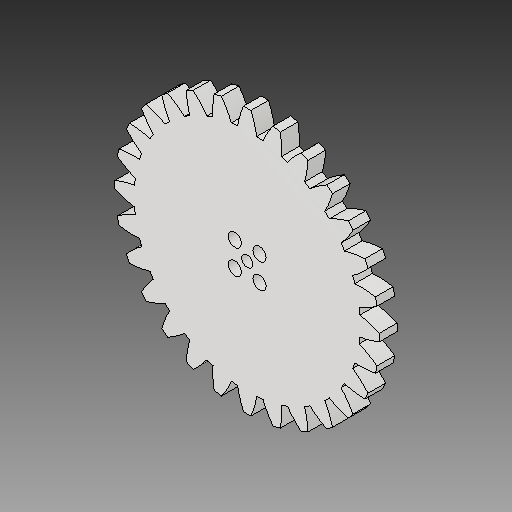
# Autodesk Inventor part: z28ギア(インベンター)
Saved by Autodesk Inventor 2019 (Build 230136000, 136)
## iProperties
Created: 2019-10-30
Part Number: z28ギア(インベンター)
Material: アセタール樹脂、白
Document SubType Name: Modeling
Designer: tanjihayato
Density: 1.425 g/cm^3
Appearance: 滑らか - 白
Mass: 13.7904 g
Surface Area: 64.1829 cm^2
Volume: 9.6775 cm^3
Author: tanjihayato
Autodesk Inventor part; units mm, degrees
ref_plane "YZ Plane" through (0, 0, 0) normal (1, 0, 0) x (0, 1, 0)
ref_plane "XZ Plane" through (0, 0, 0) normal (0, 1, 0) x (-1, 0, 0)
ref_plane "XY Plane" through (0, 0, 0) normal (0, 0, 1) x (1, 0, 0)
sketch "スケッチ1" plane through (0, 0, 0) normal (0, 0, 1) x (1, 0, 0)
  circle A0 centre (0, 0) radius 30
  circle A1 centre (0, 0) radius 8 construction
  circle A2 centre (0, 0) radius 6 construction
  circle A3 centre (0, 0) radius 1.25
  circle A4 centre (-2.8, -2.8) radius 1.5
  circle A5 centre (-2.8, 2.8) radius 1.5
  circle A6 centre (2.8, 2.8) radius 1.5
  circle A7 centre (2.8, -2.8) radius 1.5
  circle A8 centre (0, 0) radius 6 construction
  dimension "d0" = 60
  dimension "d1" = 16
  dimension "d2" = 12
  constraints: 9 centre point, 3 coincident, 5 other
  measures "d0" diameter of A0
  measures "d1" diameter of A1
  measures "d2" diameter of A2
extrude "押し出し1" add sketch "スケッチ1" along normal blind 4
spur gear teeth "平歯車1" teeth 28 pitch diameter 56 tip diameter 60 root diameter 51.2 face width 4 trims to tip circle yes start plane through (0, 0, 4) normal (0, 0, 1) x (1, 0, 0)
